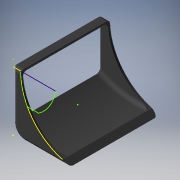
# Autodesk Inventor part: Plow
Saved by Autodesk Inventor 2019 (Build 230136000, 136)
## iProperties
Created: 2019-02-18
Part Number: Plow
Material: Generic
Document SubType Name: Modeling
Designer: Tesler
Density: 1 g/cm^3
Appearance: Default
Author: Tesler
Autodesk Inventor part; units mm, degrees
ref_plane "YZ Plane" through (0, 0, 0) normal (1, 0, 0) x (0, 1, 0)
ref_plane "XZ Plane" through (0, 0, 0) normal (0, 1, 0) x (-1, 0, 0)
ref_plane "XY Plane" through (0, 0, 0) normal (0, 0, 1) x (1, 0, 0)
sketch "Sketch1" plane through (0, 0, 0) normal (0, 0, 1) x (1, 0, 0)
  line L0 (0, 0) -> (0, 101.6)
  line L1 (0, 0) -> (95.25, 0)
  line L2 (95.25, 0) -> (84.2515, 6.35)
  line L3 (95.25, 0) -> (107.95, 0) construction
  line L4 (0, 101.6) -> (12.7, 101.6)
  arc A0 (12.7, 101.6) -> (84.2515, 6.35) centre (110.0717, 100.2457) ccw
  dimension "d0" = 101.6
  dimension "d14" = 12.7
  dimension "d15" = 150
  dimension "d16" = 12.7
  dimension "d28" = 95.25
  dimension "d48" = 97.3812
  constraints: 10 end point, 3 horizontal, 2 point on circle, 1 centre point, 1 equal length, 1 vertical
  measures "d0" distance of L0.start L0.end
  measures "d14" distance of L1.end L2.end
  measures "d15" angle of L3 L2
  measures "d16" distance of L0.end L4.end
  measures "d28" distance of L0.start L1.end
  measures "d48" radius of A0
extrude "Extrusion5" add sketch "Sketch1" along normal blind 152.4
sketch "Sketch5" plane through (0, 0, 0) normal (-1, 0, 0) x (0, 0, 1)
  line L0 (3.81, 97.79) -> (148.59, 97.79)
  line L1 (148.59, 97.79) -> (148.59, 3.175)
  line L2 (148.59, 3.175) -> (3.81, 3.175)
  line L3 (3.81, 3.175) -> (3.81, 97.79)
  line L4 (0, 101.6) -> (152.4, 101.6) projected
  line L5 (0, 0) -> (0, 101.6) projected
  line L6 (0, 0) -> (152.4, 0) projected
  line L7 (152.4, 101.6) -> (152.4, 0) projected
  dimension "d37" = 3.81
  dimension "d38" = 3.81
  dimension "d39" = 3.175
  dimension "d40" = 3.81
  constraints: 8 end point, 2 parallel, 1 horizontal, 1 perpendicular
  measures "d37" distance between parallel lines of L4 L0
  measures "d38" distance between parallel lines of L5 L3
  measures "d39" distance between parallel lines of L6 L2
  measures "d40" distance between parallel lines of L7 L1
extrude "Extrusion6" cut sketch "Sketch5" against normal blind 101.6 contours L0 L1 L2 L3
fillet "Fillet3" radius 19.05 1 edges at (0, 0, 76.2)
sketch "Sketch6" plane through (0, 97.79, 3.81) normal (0, 0, 1) x (1, 0, 0)
  arc A0 (0, -78.74) -> (19.05, -97.79) centre (19.05, -78.74) ccw projected
  arc A1 (12.7, 3.81) -> (84.2515, -91.44) centre (77.4018, 0.6973) ccw projected
  arc A2 (0, -78.74) -> (84.2515, -91.44) centre (63.4925, 56.6564) ccw
  arc A3 (0, -78.74) -> (19.05, -97.79) centre (19.05, -78.74) ccw
  line L0 (95.25, -97.79) -> (19.05, -97.79) projected
  line L1 (84.2515, -91.44) -> (95.25, -97.79) projected
  line L2 (19.05, -97.79) -> (95.25, -97.79)
  line L3 (95.25, -97.79) -> (84.2515, -91.44)
  point P0 (0, -97.79)
  dimension "d44" = 149.5443
  constraints: 4 end point, 4 point on circle, 2 centre point, 2 concentric, 1 collinear, 1 horizontal, 1 other
  measures "d44" radius of A2
extrude "Extrusion7" add sketch "Sketch6" along normal up to next
fillet "Fillet4" radius 6.35 12 edges at (41.2021, 6.5727, 148.59) (41.2021, 6.5727, 3.81) (6.3608, 97.79, 148.59) (6.35, 101.6, 152.4) (6.35, 101.6, 0) (6.3608, 97.79, 3.81) (5.5796, 5.5796, 152.4) (0, 60.325, 152.4) (57.15, 0, 152.4) (5.5796, 5.5796, 0) (0, 60.325, 0) (57.15, 0, 0)
sketch "Sketch7" plane through (0, 0, 152.4) normal (0, 0, 1) x (1, 0, 0)
  arc A0 (12.8188, 95.25) -> (84.2515, 6.35) centre (110.0717, 100.2457) ccw projected
  line L0 (12.7, 101.6) -> (0, 101.6) projected
  line L1 (12.7, 101.6) -> (72.04, 101.6)
  arc A1 (13.0895, 91.44) -> (70.1837, 11.4086) centre (110.0717, 100.2457) ccw projected
  arc A2 (12.7, 101.6) -> (24.1017, 54.5046) centre (110.0717, 100.2457) ccw
  line L2 (43.3863, 54.5046) -> (24.1017, 54.5046)
  arc A3 (43.3863, 54.5046) -> (72.04, 101.6) centre (0.6549, 112.7676) ccw
  point P0 (0, 0)
  constraints: 4 end point, 4 point on circle, 2 centre point, 2 horizontal, 1 other
body "Solid2"
